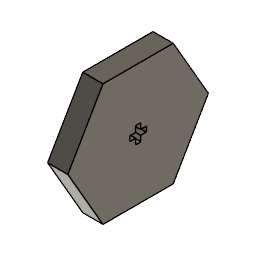
Hexagon cap Big (Autodesk Fusion 360 design; units mm, degrees)
part number: 2026-06-06-23-04-54-511
Autodesk Fusion 360 part; units mm, degrees
sketch "Sketch1" plane through (0, 0, 0) normal (1, 0, 0) x (0, 1, 0)
  line L0 (0.15, 0.15) -> (0.15, 0.477)
  line L1 (0.15, 0.15) -> (0.477, 0.15)
  line L2 (0.15, -0.15) -> (0.477, -0.15)
  line L3 (-0.15, 0.15) -> (-0.15, 0.477)
  line L4 (-0.15, 0.15) -> (-0.477, 0.15)
  line L5 (-0.15, -0.15) -> (-0.15, -0.477)
  line L6 (-0.15, -0.15) -> (-0.477, -0.15)
  line L7 (0.15, -0.15) -> (0.15, -0.477)
  arc A0 (0.477, -0.15) -> (0.477, 0.15) centre (0, 0) ccw
  arc A1 (-0.15, -0.477) -> (0.15, -0.477) centre (0, 0) ccw
  arc A2 (0.15, 0.477) -> (-0.15, 0.477) centre (0, 0) ccw
  arc A3 (-0.477, 0.15) -> (-0.477, -0.15) centre (0, 0) ccw
  line L8 (-2.0785, 3.6) -> (-4.1569, 0)
  line L9 (-4.1569, 0) -> (-2.0785, -3.6)
  line L10 (-2.0785, -3.6) -> (2.0785, -3.6)
  line L11 (2.0785, -3.6) -> (4.1569, 0)
  line L12 (4.1569, 0) -> (2.0785, 3.6)
  line L13 (2.0785, 3.6) -> (-2.0785, 3.6)
  dimension "d6" = 0.3
  dimension "d10" = 3.6
  constraint coincident A0.centre A1.centre
  constraint perpendicular L0 L1
  constraint concentric A0 A2
  constraint concentric A1 A3
  constraint concentric A2 A3
  measures "d6" distance of L0.start L2.start
  measures "d10" distance of A0.centre L13
extrude "Extrude1" add sketch "Sketch1" along normal blind 1.2
fillet "Fillet1" radius 0.1 12 edges at (0, -0.3135, -0.15) (0, -0.15, -0.3135) (0, 0, -0.5) (0, 0.15, -0.3135) (0, 0.3135, -0.15) (0, 0.5, 0) (0, 0.3135, 0.15) (0, 0.15, 0.3135) (0, 0, 0.5) (0, -0.15, 0.3135) (0, -0.3135, 0.15) (0, -0.5, 0)
